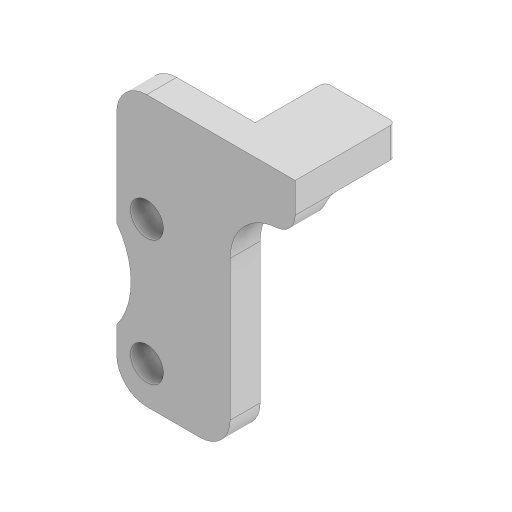
# Autodesk Inventor part: Beam breaker
Saved by Autodesk Inventor 2023 (Build 270158000, 158)
## iProperties
Created: 2026-05-18
Part Number: Beam breaker
Material: Generic
Document SubType Name: Modeling
Designer: ferrerx
Density: 1 g/cm^3
Appearance: Default
Author: ferrerx
Autodesk Inventor part; units mm, degrees
ref_plane "YZ Plane" through (0, 0, 0) normal (1, 0, 0) x (0, 1, 0)
ref_plane "XZ Plane" through (0, 0, 0) normal (0, 1, 0) x (-1, 0, 0)
ref_plane "XY Plane" through (0, 0, 0) normal (0, 0, 1) x (1, 0, 0)
sketch "Sketch1" plane through (0, 0, 0) normal (0, 0, 1) x (1, 0, 0)
  line L0 (0, 12) -> (11.3374, 12)
  line L1 (11.3374, 12) -> (11.3374, -10)
  line L2 (11.3374, -10) -> (0, -10)
  line L3 (0, -10) -> (0, 12)
  line L4 (3.0233, 0) -> (3.0233, 6.25) construction
  circle A0 centre (3.0233, 6.25) radius 1.65
  line L5 (3.0233, 0) -> (0, 0) construction
  circle A1 centre (3.0233, -6.25) radius 1.65
  circle A2 centre (-6.0697, 0) radius 7.5
  point P0 (0, 4.4056)
  point P1 (0, -4.4056)
  dimension "d0" = 3.3
  dimension "d1" = 6.25
  dimension "d2" = 11.3375
  dimension "d3" = 9.093
  dimension "d4" = 15
  dimension "d8" = 12
  dimension "d9" = 10
  constraints: 12 end point, 3 centre point, 2 horizontal, 2 parallel, 1 coincident, 1 perpendicular, 1 symmetric about line, 1 vertical, 1 other
  measures "d0" diameter of A0
  measures "d1" distance of L4.start L4.end
  measures "d2" distance of L0.start L0.end
  measures "d3" distance of A2.centre L4.start
  measures "d4" diameter of A2
  measures "d8" distance between parallel lines of L5 L0
  measures "d9" distance between parallel lines of L5 L2
extrude "Extrusion1" add sketch "Sketch1" along normal blind 3 contours L0 L1 L2 L3 A2
sketch "Sketch2" plane through (0, 0, 0) normal (0, 0, -1) x (-1, 0, 0)
  line L0 (-11.3374, 12) -> (0, 12) projected
  line L1 (0, 12) -> (-17.8374, 12)
  line L2 (-17.8374, 12) -> (-17.8374, 17)
  line L3 (-17.8374, 17) -> (0, 17)
  line L4 (0, 17) -> (0, 12)
  line L5 (-11.3374, -10) -> (-11.3374, 12) projected
  point P0 (0, 0)
  dimension "d10" = 6.5
  dimension "d11" = 5
  constraints: 8 end point, 2 parallel, 1 horizontal, 1 perpendicular
  measures "d10" distance between parallel lines of L5 L2
  measures "d11" distance of L1.end L2.end
extrude "Extrusion2" add sketch "Sketch2" against normal blind 3
sketch "Sketch3" plane through (0, 0, 0) normal (0, 0, -1) x (-1, 0, 0)
  line L0 (-17.8374, 17) -> (0, 17) projected
  line L1 (-17.8374, 17) -> (-10.8374, 17)
  line L2 (-10.8374, 17) -> (-10.8374, 14)
  line L3 (-10.8374, 14) -> (-17.8374, 14)
  line L4 (-17.8374, 14) -> (-17.8374, 17)
  point P0 (0, 0)
  dimension "d14" = 3
  dimension "d15" = 7
  constraints: 8 end point, 2 parallel, 1 horizontal, 1 perpendicular
  measures "d14" distance between parallel lines of L0 L3
  measures "d15" distance of L2.end L3.end
extrude "Extrusion3" add sketch "Sketch3" along normal blind 7
fillet "Fillet1" radius 3 3 edges at (11.3374, -10, 1.5) (0, -10, 1.5) (0, 17, 1.5)
fillet "Fillet2" radius 5 1 edges at (11.3374, 12, 1.5)
fillet "Fillet3" radius 2 1 edges at (17.8374, 12, 1.5)
fillet "Fillet4" radius 1 1 edges at (14.3374, 14, 0)
fillet "Fillet5" radius 0.5 2 edges at (17.8374, 15.5, -7) (10.8374, 15.5, -7)
body "Solid1"
